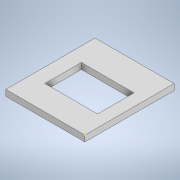
# Autodesk Inventor part: SpeakerSurfaceFinal
Saved by Autodesk Inventor 2020 (Build 240168000, 168)
## iProperties
Created: 2022-02-15
Part Number: SpeakerSurfaceFinal
Material: Generic
Document SubType Name: Modeling
Designer: iss
Density: 1 g/cm^3
Appearance: Default
Author: iss
Autodesk Inventor part; units mm, degrees
ref_plane "YZ Plane" through (0, 0, 0) normal (1, 0, 0) x (0, 1, 0)
ref_plane "XZ Plane" through (0, 0, 0) normal (0, 1, 0) x (-1, 0, 0)
ref_plane "XY Plane" through (0, 0, 0) normal (0, 0, 1) x (1, 0, 0)
sketch "Sketch1" plane through (0, 0, 0) normal (0, 1, 0) x (-1, 0, 0)
  line L0 (0, 0) -> (39, 0)
  line L1 (39, 0) -> (39, -44)
  line L2 (39, -44) -> (0, -44)
  line L3 (0, -44) -> (0, 0)
  dimension "d0" = 39
  dimension "d1" = 44
  constraints: 8 end point, 2 parallel, 1 horizontal, 1 perpendicular
  measures "d0" distance of L1.end L2.end
  measures "d1" distance of L0.end L1.end
extrude "Extrusion1" add sketch "Sketch1" along normal blind 3
sketch "Sketch2" plane through (0, 3, 0) normal (0, 1, 0) x (1, 0, 0)
  line L0 (-31.9002, 12.1338) -> (-5.9002, 12.1338)
  line L1 (-5.9002, 12.1338) -> (-5.9002, 30.1338)
  line L2 (-5.9002, 30.1338) -> (-31.9002, 30.1338)
  line L3 (-31.9002, 30.1338) -> (-31.9002, 12.1338)
  point P0 (0, 0)
  dimension "d4" = 26
  dimension "d5" = 18
  constraints: 8 end point, 2 parallel, 1 horizontal, 1 perpendicular
  measures "d4" distance of L2.end L1.end
  measures "d5" distance of L1.end L0.end
extrude "Extrusion2" cut sketch "Sketch2" against normal blind 3.25
sketch "Sketch3" plane through (0, 3, 0) normal (0, 1, 0) x (1, 0, 0)
  point P0 (0, 0)
body "Solid1"
